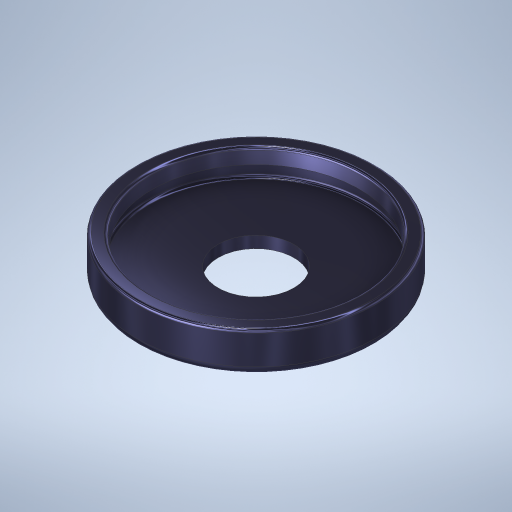
# Autodesk Inventor part: Shock Cartridge Cover
Saved by Autodesk Inventor 2023.1 (Build 271208000, 208)
## iProperties
Created: 2019-11-30
Part Number: Shock Cartridge Cover
Material: Generic
Document SubType Name: Modeling
Designer: Jopa
Density: 1 g/cm^3
Appearance: Default
Author: Jopa
Autodesk Inventor part; units mm, degrees
ref_plane "YZ Plane" through (0, 0, 0) normal (1, 0, 0) x (0, 1, 0)
ref_plane "XZ Plane" through (0, 0, 0) normal (0, 1, 0) x (-1, 0, 0)
ref_plane "XY Plane" through (0, 0, 0) normal (0, 0, 1) x (1, 0, 0)
sketch "Sketch1" plane through (0, 0, 0) normal (0, 0, 1) x (1, 0, 0)
  line L0 (-1.0414, 0) -> (6.2484, 0) construction
  line L1 (0, -0.3556) -> (0, 2.1336) construction
  line L2 (1.651, 0) -> (5.207, 0)
  line L3 (5.207, 0) -> (5.207, 1.778)
  line L4 (5.207, 1.778) -> (4.572, 1.778)
  line L5 (4.572, 1.778) -> (4.5189, 1.143)
  line L6 (4.5189, 1.143) -> (4.7625, 1.143)
  line L7 (4.7625, 1.143) -> (4.7625, 0.508)
  line L8 (4.7625, 0.508) -> (1.651, 0.508)
  line L9 (1.651, 0.508) -> (1.651, 0)
  point P0 (0, 0)
  dimension "d0" = 3.302
  dimension "d1" = 10.414
  dimension "d2" = 1.778
  dimension "d3" = 0.635
  dimension "d4" = 9.0378
  dimension "d5" = 9.525
  dimension "d6" = 0.508
  dimension "d7" = 0.635
  constraints: 16 end point, 3 perpendicular, 2 point on line, 1 horizontal, 1 parallel, 1 vertical
  measures "d0" diameter of L2.start L1
  measures "d1" diameter of L3 L1
  measures "d2" distance of L2.end L3.end
  measures "d3" distance of L3.end L4.end
  measures "d4" diameter of L5.end L1
  measures "d5" diameter of L7 L1
  measures "d6" distance of L8.end L2.start
  measures "d7" distance between parallel lines of L4 L6
revolve "Revolution1" add sketch "Sketch1" angle 360 about axis through (0, -10, 0) along (0, 1, 0)
fillet "Fillet1" radius 0.381 1 edges at (-5.207, 0, 0)
fillet "Fillet2" radius 0.127 3 edges at (-5.207, 1.778, 0) (-4.572, 1.778, 0) (-4.7625, 0.508, 0)
equation "\"d7\" = d3"
body "Solid1"
